Autodesk Inventor part; units mm, degrees
(part 2 of 3)
  measures "d1135" distance of L2.end L36.start
  measures "d1140" distance of L13.end A26.centre
  measures "d1141" distance from line of A2.centre L178
  measures "d1142" distance of L20.end L181.end
  measures "d1145" distance of A4.centre A28.centre
extrude "Extrusion27" add sketch "Sketch20" against normal blind 0.025 contours A0 L0 L8 A1 L7 L4 | A1 L32 L31 L30 | L41 A7 L40 L13 A6 | L9 A2 L10 A3 | A3 L177 L178 L179 | L45 L44 L43 A7 | L54 A9 L53 L13 A8 | L11 A38 A39 | A39 L402 L401 L400 | L58 L57 L56 A9 | L11 A36 L247 A37 L248 | A37 L253 L254 L255 | L67 A11 L66 L13 A10 | L71 L70 L69 A11 | L11 A41 L257 A40 L264 | A40 L257 L262 L266 | L80 A13 L79 L13 A12 | L84 L83 L82 A13 | L11 A43 L270 A42 L277 | A42 L270 L275 L279 | L93 A15 L92 L13 A14 | L97 L96 L95 A15 | L11 A45 L283 A44 L290 | A44 L283 L288 L292 | L106 A17 L105 L13 A16 | L110 L109 L108 A17 | L11 A47 L296 A46 L303 | A46 L296 L301 L305 | L119 A19 L118 L13 A18 | L123 L122 L121 A19 | L11 A49 L309 A48 L316 | A48 L309 L314 L318 | L132 A21 L131 L13 A20 | L136 L135 L134 A21 | L11 A51 L322 A50 L329 | A50 L322 L327 L331 | L145 A23 L144 L13 A22 | L149 L148 L147 A23 | L11 A53 L335 A52 L342 | A52 L335 L340 L344 | L158 A25 L157 L13 A24 | L162 L161 L160 A25 | L11 A55 L348 A54 L355 | A54 L348 L353 L357 | L171 A27 L170 L13 A26 | L175 L174 L173 A27 | L11 A57 L361 A56 L368 | A56 L361 L366 L370 | L22 A5 L28 L14 A4 | L182 L181 L180 A5 | L11 A59 L374 A58 L381 | A58 L374 L379 L383 | L186 A29 L192 L14 A28 | L196 L195 L194 A29 | L11 A61 L387 A60 L394 | A60 L387 L392 L396 | L200 A31 L206 L14 A30 | L210 L209 L208 A31 | L14 A34 L228 A35 L234 | A35 L238 L237 L236 | L214 A33 L220 L14 A32 | L224 L223 L222 A33
extrude "Extrusion28" add sketch "Sketch20" along normal blind 0.625 contours A0 L0 L8 A1 L7 L4 | L41 A7 L40 L13 A6 | L9 A2 L10 A3 | L54 A9 L53 L13 A8 | L11 A38 A39 | L11 A36 L247 A37 L248 | L67 A11 L66 L13 A10 | L11 A41 L257 A40 L264 | L80 A13 L79 L13 A12 | L11 A43 L270 A42 L277 | L93 A15 L92 L13 A14 | L11 A45 L283 A44 L290 | L106 A17 L105 L13 A16 | L11 A47 L296 A46 L303 | L119 A19 L118 L13 A18 | L11 A49 L309 A48 L316 | L132 A21 L131 L13 A20 | L11 A51 L322 A50 L329 | L145 A23 L144 L13 A22 | L11 A53 L335 A52 L342 | L158 A25 L157 L13 A24 | L11 A55 L348 A54 L355 | L171 A27 L170 L13 A26 | L11 A57 L361 A56 L368 | L22 A5 L28 L14 A4 | L11 A59 L374 A58 L381 | L186 A29 L192 L14 A28 | L11 A61 L387 A60 L394 | L200 A31 L206 L14 A30 | L14 A34 L228 A35 L234 | L214 A33 L220 L14 A32
sketch "Sketch15" plane through (0, 0, 0.6) normal (0, 0, 1) x (1, 0, 0)
  line L0 (-6.2, -4) -> (1.6, -4)
  line L1 (1.6, -4) -> (1.6, 4)
  line L2 (1.6, 4) -> (-6.2, 4)
  line L3 (-6.2, 4) -> (-6.2, -4)
  line L4 (-6.2, -4) -> (1.6, 4) construction
  line L5 (1.6, -4) -> (-6.2, 4) construction
  line L6 (-6.5, 4.3) -> (1.9, 4.3)
  line L7 (1.9, 4.3) -> (1.9, -4.3)
  line L8 (1.9, -4.3) -> (-6.5, -4.3)
  line L9 (-6.5, -4.3) -> (-6.5, 4.3)
  line L10 (-6.2, 4) -> (-6.5, 4)
  line L11 (-6.5, 4) -> (-6.5, 4.3)
  line L12 (-6.5, 4.3) -> (-6.2, 4.3)
  line L13 (-6.2, 4.3) -> (-6.2, 4)
  line L14 (1.6, 4) -> (1.9, 4)
  line L15 (1.9, 4) -> (1.9, 4.3)
  line L16 (1.9, 4.3) -> (1.6, 4.3)
  line L17 (1.6, 4.3) -> (1.6, 4)
  line L18 (1.6, -4) -> (1.9, -4)
  line L19 (1.9, -4) -> (1.9, -4.3)
  line L20 (1.9, -4.3) -> (1.6, -4.3)
  line L21 (1.6, -4.3) -> (1.6, -4)
  line L22 (-6.5, -4.3) -> (-6.2, -4.3)
  line L23 (-6.2, -4.3) -> (-6.2, -4)
  line L24 (-6.2, -4) -> (-6.5, -4)
  line L25 (-6.5, -4) -> (-6.5, -4.3)
  line L26 (-6.975, 4.775) -> (-6.975, 2.27) projected
  line L27 (-6.47, 4.775) -> (-6.975, 4.775) projected
  line L28 (-6.2975, -4.1) -> (1.6975, -4.1)
  line L29 (1.6975, -4.1) -> (1.6975, 4.1)
  line L30 (1.6975, 4.1) -> (-6.2975, 4.1)
  line L31 (-6.2975, 4.1) -> (-6.2975, -4.1)
  line L32 (-6.2975, -4.1) -> (1.6975, 4.1) construction
  line L33 (1.6975, -4.1) -> (-6.2975, 4.1) construction
  arc A0 (-6.975, -0.27) -> (-6.975, 0.27) centre (-6.975, 0) ccw projected
  point P0 (-2.3, 0)
  point P1 (-2.3, 0)
  point P2 (-6.705, 0)
  dimension "d952" = 7.8
  dimension "d953" = 8
  dimension "d954" = 0.3
  dimension "d961" = 0.475
  dimension "d962" = 0.475
  dimension "d966" = 0.1
  constraints: 64 end point, 14 parallel, 7 perpendicular, 6 horizontal, 5 midpoint, 1 horizontal alignment, 1 point on circle, 1 point on line, 3 other
  measures "d952" distance of L2.end L1.end
  measures "d953" distance of L1.end L0.end
  measures "d954" distance between parallel lines of L2 L6
  measures "d961" distance between parallel lines of L9 L26
  measures "d962" distance between parallel lines of L27 L6
  measures "d966" distance between parallel lines of L30 L2
extrude "Extrusion20" add sketch "Sketch15" along normal blind 1.55
fillet "Fillet4" radius 0.3 4 edges at (1.9, 0, 2.15) (-2.3, -4.3, 2.15) (-2.3, 4.3, 2.15) (-6.5, 0, 2.15)
extrude "Extrusion22" cut sketch "Sketch15" along normal through all contours L23 L28 L31 L24 | L18 L29 L28 L21 | L10 L31 L30 L13 | L23 L8 L9 L24 L31 L28 | L17 L30 L29 L14 | L18 L7 L8 L21 L28 L29 | L10 L9 L6 L13 L30 L31 | L29 L30 L17 L6 L7 L14
extrude "Extrusion23" cut sketch "Sketch15" along normal blind 1.4 contours L3 L2 L1 L0 | L24 L31 L10 L3 | L0 L21 L28 L23 | L23 L28 L31 L24 | L1 L14 L29 L18 | L18 L29 L28 L21 | L13 L30 L17 L2 | L10 L31 L30 L13 | L17 L30 L29 L14
fillet "Fillet5" radius 0.3 4 edges at (-2.3, -4.1, 2) (-6.2975, 0, 2) (-2.3, 4.1, 2) (1.6975, 0, 2)
extrude "Extrusion24" cut sketch "Sketch15" along normal blind 0.1 contours L3 L2 L1 L0 | L24 L31 L10 L3 | L0 L21 L28 L23 | L23 L28 L31 L24 | L1 L14 L29 L18 | L18 L29 L28 L21 | L13 L30 L17 L2 | L10 L31 L30 L13 | L28 L21 L8 L23 | L24 L9 L10 L31 | L17 L30 L29 L14 | L29 L14 L7 L18 | L13 L6 L17 L30
sketch "Sketch16" plane through (0, 0, 2.15) normal (0, 0, 1) x (1, 0, 0)
  line L0 (0.9007, -3.777) -> (-5.4993, -3.777)
  line L1 (-5.9993, -3.277) -> (-5.9993, 3.123)
  line L2 (-5.4993, 3.623) -> (0.9007, 3.623)
  line L3 (1.4007, 3.123) -> (1.4007, -3.277)
  line L4 (1.4007, -3.777) -> (-5.9993, 3.623) construction
  line L5 (-5.9993, -3.777) -> (1.4007, 3.623) construction
  arc A0 (-5.4993, 3.623) -> (-5.9993, 3.123) centre (-5.4993, 3.123) ccw
  arc A1 (1.4007, 3.123) -> (0.9007, 3.623) centre (0.9007, 3.123) ccw
  arc A2 (0.9007, -3.777) -> (1.4007, -3.277) centre (0.9007, -3.277) ccw
  arc A3 (-5.9993, -3.277) -> (-5.4993, -3.777) centre (-5.4993, -3.277) ccw
  point P0 (-2.2993, -0.077)
  point P1 (-2.2993, -0.077)
  dimension "d957" = 7.4
  dimension "d958" = 0.5
  constraints: 12 end point, 8 point on circle, 8 point on line, 8 tangent, 4 centre point, 3 equal radius, 2 parallel, 2 perpendicular, 1 coincident, 1 horizontal, 1 midpoint
  measures "d957" distance of L4.end L5.end
  measures "d958" radius of A0
extrude "Extrusion21" add sketch "Sketch16" along normal blind 0.1
sketch "Sketch18" plane through (0, 0, 2.25) normal (0, 0, 1) x (1, 0, 0)
  line L0 (0.9007, -3.777) -> (-5.4993, -3.777)
  line L1 (-5.9993, -3.277) -> (-5.9993, 3.123)
  line L2 (-5.4993, 3.623) -> (0.9007, 3.623)
  line L3 (1.4007, 3.123) -> (1.4007, -3.277)
  line L4 (1.4007, -3.777) -> (-5.9993, 3.623) construction
  line L5 (-5.9993, -3.777) -> (1.4007, 3.623) construction
  arc A0 (-5.4993, 3.623) -> (-5.9993, 3.123) centre (-5.4993, 3.123) ccw
  arc A1 (1.4007, 3.123) -> (0.9007, 3.623) centre (0.9007, 3.123) ccw
  arc A2 (0.9007, -3.777) -> (1.4007, -3.277) centre (0.9007, -3.277) ccw
  arc A3 (-5.9993, -3.277) -> (-5.4993, -3.777) centre (-5.4993, -3.277) ccw
  line L6 (-5.9993, -2.3578) -> (-4.5801, -3.777)
  line L7 (1.4007, -3.277) -> (1.4007, 3.123) projected
  line L8 (0.9007, 3.623) -> (-5.4993, 3.623) projected
  point P0 (-2.2993, -0.077)
  point P1 (-2.2993, -0.077)
  dimension "d972" = 7.4
  dimension "d973" = 0.5
  dimension "d976" = 45
  constraints: 14 end point, 10 point on line, 8 point on circle, 8 tangent, 4 centre point, 3 equal radius, 2 collinear, 2 parallel, 2 perpendicular, 1 coincident, 1 horizontal, 1 midpoint
  measures "d972" distance of L4.end L5.end
  measures "d973" radius of A0
  measures "d976" angle of L1 L6
extrude "Extrusion25" add sketch "Sketch18" along normal blind 0.001 contours L0 A3 L1 L6
sketch "Sketch17" plane through (0, 0, 2.25) normal (0, 0, 1) x (1, 0, 0)
  line L0 (-2.3072, -0.8881) -> (-2.4609, -0.8881)
  line L1 (-2.3072, -0.7289) -> (-2.3072, -0.8881)
  line L2 (-2.4609, -1.0504) -> (-2.1407, -1.0504)
  line L3 (-2.4668, -0.7289) -> (-2.3072, -0.7289)
  line L4 (-2.7903, -0.5636) -> (-2.7903, -0.7289)
  line L5 (-2.4668, -0.5636) -> (-2.4668, -0.7289)
  line L6 (-2.63, -0.5636) -> (-2.7903, -0.5636)
  line L7 (-2.63, -0.4013) -> (-2.7903, -0.4013)
  line L8 (-2.63, -0.4013) -> (-2.63, -0.5636)
  line L9 (-2.3072, -0.7289) -> (-2.3072, -0.5636)
  line L10 (-2.1407, -0.7289) -> (-2.3072, -0.7289)
  line L11 (-2.3072, -0.5636) -> (-2.1407, -0.5636)
  line L12 (-2.3072, -0.4013) -> (-2.4684, -0.4013)
  line L13 (-2.3072, -0.4013) -> (-2.3072, -0.5636)
  line L14 (-2.3072, -0.5636) -> (-2.4668, -0.5636)
  line L15 (-2.3037, -1.207) -> (-2.3037, -1.3643)
  line L16 (-4.4057, -1.2114) -> (-4.4057, -0.8881)
  line L17 (-4.0783, -1.2114) -> (-4.2447, -1.2114)
  line L18 (-4.5693, -1.2114) -> (-4.4057, -1.2114)
  line L19 (-4.2447, -1.2114) -> (-4.2447, -1.3643)
  line L20 (-4.2447, -1.3643) -> (-4.4057, -1.3643)
  line L21 (-4.0783, -1.3643) -> (-4.0783, -1.2114)
  line L22 (-3.9152, -1.3643) -> (-4.0783, -1.3643)
  line L23 (-4.2447, -1.5323) -> (-3.9212, -1.5323)
  line L24 (-3.9212, -1.5323) -> (-3.9212, -1.6965)
  line L25 (-4.2447, -1.6965) -> (-4.2447, -1.5323)
  line L26 (-4.5693, -1.6901) -> (-4.5693, -1.2114)
  line L27 (-4.4057, -1.3643) -> (-4.4057, -1.6901)
  line L28 (-4.4057, -1.6901) -> (-4.5693, -1.6901)
  line L29 (-3.2789, -0.8881) -> (-3.7606, -0.8881)
  line L30 (-3.6008, -1.0498) -> (-3.2789, -1.0498)
  line L31 (-3.6008, -1.2061) -> (-3.6008, -1.0498)
  line L32 (-3.2789, -1.2061) -> (-3.6008, -1.2061)
  line L33 (-3.7606, -1.2061) -> (-3.6008, -1.2061)
  line L34 (-3.7606, -0.8881) -> (-3.7606, -1.2061)
  line L35 (-3.2789, -1.3643) -> (-3.2789, -1.2061)
  line L36 (-3.6008, -1.3643) -> (-3.4396, -1.3643)
  line L37 (-3.6008, -1.2061) -> (-3.6008, -1.3643)
  line L38 (-3.9152, -0.8881) -> (-3.9152, -1.3643)
  line L39 (-3.4396, -1.3643) -> (-3.4396, -1.5272)
  line L40 (-3.439, -0.7259) -> (-3.6002, -0.7259)
  line L41 (-3.2789, -1.0498) -> (-3.2789, -0.8881)
  line L42 (-3.1151, -1.0498) -> (-3.2789, -1.0498)
  line L43 (-3.1151, -0.8881) -> (-3.1151, -1.0498)
  line L44 (-2.9507, -0.8881) -> (-3.1151, -0.8881)
  line L45 (-3.2789, -1.0498) -> (-3.2789, -1.2061)
  line L46 (-1.8231, -0.8881) -> (-1.6598, -0.8881)
  line L47 (-1.4972, -1.0504) -> (-1.8231, -1.0504)
  line L48 (-1.9819, -0.8881) -> (-2.1407, -0.8881)
  line L49 (-2.1407, -0.7289) -> (-2.1407, -0.8881)
  line L50 (-1.8231, -1.0504) -> (-1.8231, -0.8881)
  line L51 (-2.1407, -1.0504) -> (-2.1407, -1.207)
  line L52 (-1.9819, -1.207) -> (-1.9819, -0.8881)
  line L53 (-1.8231, -1.215) -> (-1.6598, -1.215)
  line L54 (-1.6598, -0.8881) -> (-1.6598, -0.7289)
  line L55 (-3.9212, -0.4013) -> (-3.9212, -0.5636)
  line L56 (-3.9212, -0.5636) -> (-4.0807, -0.5636)
  line L57 (-4.2425, -0.4013) -> (-3.9212, -0.4013)
  line L58 (-4.2447, -0.4013) -> (-4.4057, -0.4013)
  line L59 (-4.5665, -0.5636) -> (-4.2425, -0.5636)
  line L60 (-4.5665, -0.7259) -> (-4.5665, -0.5636)
  line L61 (-4.2395, -0.7259) -> (-4.5665, -0.7259)
  line L62 (-4.0807, -0.8881) -> (-3.9152, -0.8881)
  line L63 (-4.4057, -0.8881) -> (-4.2395, -0.8881)
  line L64 (-4.2395, -0.8881) -> (-4.2395, -0.7259)
  line L65 (-4.0807, -0.5636) -> (-4.0807, -0.8881)
  line L66 (-4.2425, -0.5636) -> (-4.2425, -0.4013)
  line L67 (-2.9501, -0.4013) -> (-2.9501, -0.7259)
  line L68 (-2.9501, -0.7259) -> (-3.1162, -0.7259)
  line L69 (-3.1162, -0.4013) -> (-2.9501, -0.4013)
  line L70 (-3.1162, -0.7259) -> (-3.1162, -0.5636)
  line L71 (-3.6002, -0.5628) -> (-3.439, -0.5628)
  line L72 (-3.6002, -0.7259) -> (-3.6002, -0.5628)
  line L73 (-3.439, -0.5628) -> (-3.439, -0.7259)
  line L74 (-3.1162, -0.5636) -> (-3.2789, -0.5636)
  line L75 (-3.2789, -0.5636) -> (-3.2789, -0.4013)
  line L76 (-3.9212, -1.6965) -> (-4.2447, -1.6965)
  line L77 (-4.2456, -2.1791) -> (-3.7554, -2.1791)
  line L78 (-4.4066, -2.0183) -> (-3.6011, -2.0183)
  line L79 (-4.2456, -2.6678) -> (-4.2456, -2.1791)
  line L80 (-4.5703, -1.8527) -> (-3.4399, -1.8527)
  line L81 (-4.4066, -2.8312) -> (-4.4066, -2.0183)
  line L82 (-3.7554, -2.1791) -> (-3.7554, -2.6678)
  line L83 (-3.7554, -2.6678) -> (-4.2456, -2.6678)
  line L84 (-4.5703, -2.982) -> (-4.5703, -1.8527)
  line L85 (-3.6011, -2.0183) -> (-3.6011, -2.8312)
  line L86 (-3.6011, -2.8312) -> (-4.4066, -2.8312)
  line L87 (-3.4399, -2.982) -> (-4.5703, -2.982)
  line L88 (-3.4399, -1.8527) -> (-3.4399, -2.982)
  line L89 (-2.7903, -0.7289) -> (-2.63, -0.7289)
  line L90 (-2.63, -0.7289) -> (-2.63, -1.207)
  line L91 (-2.9507, -1.2061) -> (-2.9507, -0.8881)
  line L92 (-2.4609, -0.8881) -> (-2.4609, -1.0504)
  line L93 (-2.9501, -1.8542) -> (-2.9501, -2.0183)
  line L94 (-2.9501, -2.1791) -> (-2.6293, -2.1791)
  line L95 (-2.7903, -1.8542) -> (-2.9501, -1.8542)
  line L96 (-2.9501, -2.0183) -> (-2.7903, -2.0183)
  line L97 (-2.7903, -2.0183) -> (-2.7903, -1.8542)
  line L98 (-2.63, -2.0183) -> (-2.63, -1.8542)
  line L99 (-2.7903, -1.6901) -> (-2.9507, -1.6901)
  line L100 (-2.7903, -1.6901) -> (-2.7903, -1.8542)
  line L101 (-2.9507, -1.5272) -> (-2.9507, -1.6901)
  line L102 (-2.7903, -1.8542) -> (-2.63, -1.8542)
  line L103 (-2.63, -1.5272) -> (-2.9507, -1.5272)
  line L104 (-2.9507, -1.8542) -> (-2.9507, -1.6901)
  line L105 (-3.2789, -1.2061) -> (-2.9507, -1.2061)
  line L106 (-3.2789, -1.3643) -> (-2.9507, -1.3643)
  line L107 (-3.7606, -1.5272) -> (-3.7606, -1.6901)
  line L108 (-3.4396, -1.5272) -> (-3.7606, -1.5272)
  line L109 (-3.7606, -1.6901) -> (-3.2789, -1.6901)
  line L110 (-3.2789, -1.5272) -> (-2.9507, -1.5272)
  line L111 (-3.2789, -1.5272) -> (-3.2789, -1.6901)
  line L112 (-3.1153, -2.0183) -> (-2.9501, -2.0183)
  line L113 (-3.1153, -1.8542) -> (-2.9507, -1.8542)
  line L114 (-2.9501, -2.0183) -> (-2.9501, -2.1791)
  line L115 (-2.9507, -1.6901) -> (-3.2789, -1.6901)
  line L116 (-3.2789, -1.6901) -> (-3.2789, -2.0183)
  line L117 (-3.1153, -2.1791) -> (-3.1153, -2.0183)
  line L118 (-3.2789, -2.0183) -> (-3.1153, -2.0183)
  line L119 (-3.1153, -2.0183) -> (-3.1153, -1.8542)
  line L120 (-1.1756, -0.4013) -> (-1.1756, -0.728)
  line L121 (-1.1766, -0.4013) -> (-1.3407, -0.4013)
  line L122 (-1.1741, -0.8881) -> (-0.5231, -0.8881)
  line L123 (-0.6864, -0.728) -> (-0.8486, -0.728)
  line L124 (-0.8486, -0.728) -> (-0.8486, -0.5636)
  line L125 (-0.8486, -0.5636) -> (-1.0117, -0.5636)
  line L126 (-0.8486, -0.5636) -> (-0.6864, -0.5636)
  line L127 (-0.6864, -0.5636) -> (-0.6864, -0.728)
  line L128 (-0.5231, -0.8881) -> (-0.5231, -0.4013)
  line L129 (-2.1407, -0.4013) -> (-2.1407, -0.5636)
  line L130 (-1.8231, -0.4013) -> (-2.1407, -0.4013)
  line L131 (-1.6598, -0.7289) -> (-1.3365, -0.7289)
  line L132 (-1.3365, -0.7289) -> (-1.3365, -0.5636)
  line L133 (-1.3365, -0.5636) -> (-1.8231, -0.5636)
  line L134 (-1.6598, -0.4013) -> (-1.8231, -0.4013)
  line L135 (-1.8231, -0.5636) -> (-1.8231, -0.4013)
  line L136 (-2.63, -1.2061) -> (-2.63, -1.3643)
  line L137 (-2.63, -1.3643) -> (-2.63, -1.5272)
  line L138 (-2.9507, -1.5272) -> (-2.9507, -1.3643)
  line L139 (-2.63, -1.3643) -> (-2.9507, -1.3643)
  line L140 (-2.9507, -1.2061) -> (-2.63, -1.2061)
  line L141 (-2.9507, -1.3643) -> (-2.9507, -1.2061)
  line L142 (-2.63, -1.207) -> (-2.3037, -1.207)
  line L143 (-2.4668, -1.3643) -> (-2.63, -1.3643)
  line L144 (-2.63, -1.8542) -> (-2.4668, -1.8542)
  line L145 (-2.4684, -1.6901) -> (-2.4684, -1.8542)
  line L146 (-2.63, -1.6901) -> (-2.4684, -1.6901)
  line L147 (-2.63, -1.8542) -> (-2.63, -1.6901)
  line L148 (-2.4684, -1.8542) -> (-2.3037, -1.8542)
  line L149 (-2.4668, -2.0183) -> (-2.63, -2.0183)
  line L150 (-2.4668, -1.8542) -> (-2.4668, -2.0183)
  line L151 (-2.6293, -2.338) -> (-2.4677, -2.338)
  line L152 (-2.6293, -2.1791) -> (-2.6293, -2.338)
  line L153 (-2.3037, -1.8542) -> (-2.3037, -2.1797)
  line L154 (-2.1407, -1.8542) -> (-1.9783, -1.8542)
  line L155 (-2.1407, -2.1797) -> (-2.1407, -1.8542)
  line L156 (-1.9783, -1.8542) -> (-1.9783, -2.1797)
  line L157 (-2.3008, -2.1797) -> (-2.4677, -2.1797)
  line L158 (-2.4677, -2.1797) -> (-2.4677, -2.338)
  line L159 (-2.3037, -2.1797) -> (-2.1407, -2.1797)
  line L160 (-2.3008, -2.338) -> (-2.3008, -2.1797)
  line L161 (-2.4677, -2.338) -> (-2.3008, -2.338)
  line L162 (-2.4677, -2.338) -> (-2.4677, -2.5032)
  line L163 (-2.4677, -2.5032) -> (-1.9776, -2.5032)
  line L164 (-1.4972, -1.6901) -> (-1.4972, -1.5272)
  line L165 (-1.4972, -1.5272) -> (-1.3365, -1.5272)
  line L166 (-1.3365, -1.5272) -> (-1.3365, -1.3643)
  line L167 (-1.3365, -1.3643) -> (-1.4972, -1.3643)
  line L168 (-1.4972, -1.3643) -> (-1.4972, -1.0504)
  line L169 (-0.3615, -0.5636) -> (-0.3615, -0.4013)
  line L170 (-0.0419, -0.5636) -> (0.1158, -0.5636)
  line L171 (-0.3615, -0.4013) -> (-0.0419, -0.4013)
  line L172 (-0.0419, -0.4013) -> (-0.0419, -0.5636)
  line L173 (-0.1998, -0.8881) -> (-0.1998, -1.0498)
  line L174 (-0.2017, -0.5636) -> (-0.3615, -0.5636)
  line L175 (-0.3615, -1.207) -> (-0.0419, -1.207)
  line L176 (-0.0419, -1.0498) -> (-0.0419, -1.207)
  line L177 (-0.2017, -0.728) -> (-0.2017, -0.5636)
  line L178 (-0.0419, -0.728) -> (-0.2017, -0.728)
  line L179 (-0.0419, -1.0498) -> (-0.1998, -1.0498)
  line L180 (-0.0419, -1.0507) -> (-0.0419, -0.728)
  line L181 (0.1158, -1.0507) -> (-0.0419, -1.0507)
  line L182 (0.1158, -0.5636) -> (0.1158, -1.0507)
  line L183 (-1.1741, -1.0498) -> (-1.1741, -0.8881)
  line L184 (-1.1756, -0.728) -> (-1.3361, -0.728)
  line L185 (-1.3361, -0.728) -> (-1.3361, -1.0498)
  line L186 (-1.0117, -1.0498) -> (-0.6878, -1.0498)
  line L187 (-1.0117, -1.207) -> (-1.0117, -1.0498)
  line L188 (-1.3361, -1.0498) -> (-1.1741, -1.0498)
  line L189 (-1.3365, -1.3643) -> (-0.3615, -1.3643)
  line L190 (-1.3365, -1.3643) -> (-1.3365, -1.207)
  line L191 (-1.3365, -1.207) -> (-1.0117, -1.207)
  line L192 (-0.6878, -1.0498) -> (-0.6878, -1.207)
  line L193 (-0.6878, -1.207) -> (-0.5231, -1.207)
  line L194 (-0.5231, -1.207) -> (-0.5231, -0.8881)
  line L195 (-0.5231, -0.8881) -> (-0.1998, -0.8881)
  line L196 (-0.3615, -1.207) -> (-0.3615, -1.3643)
  line L197 (-0.1997, -1.3643) -> (-0.3615, -1.3643)
  line L198 (0.1158, -1.3707) -> (-0.0419, -1.3707)
  line L199 (-0.0419, -1.3707) -> (-0.0419, -1.5323)
  line L200 (-0.1997, -1.5323) -> (-0.1997, -1.3643)
  line L201 (-0.0419, -1.5323) -> (-0.1997, -1.5323)
  line L202 (-0.3615, -1.3643) -> (-0.3615, -1.5323)
  line L203 (-0.3615, -1.5323) -> (-0.1997, -1.5323)
  line L204 (0.1158, -1.6965) -> (0.1158, -1.3707)
  line L205 (-0.1997, -1.6965) -> (0.1158, -1.6965)
  line L206 (-0.1997, -1.5323) -> (-0.1997, -1.6965)
  line L207 (-2.1407, -1.5322) -> (-2.4668, -1.5322)
  line L208 (-2.4668, -1.5322) -> (-2.4668, -1.3643)
  line L209 (-2.1407, -1.207) -> (-1.9819, -1.207)
  line L210 (-2.1407, -1.3643) -> (-2.1407, -1.5322)
  line L211 (-2.1407, -1.5323) -> (-1.9792, -1.5323)
  line L212 (-2.1407, -1.6965) -> (-2.1407, -1.5323)
  line L213 (-1.8231, -1.5323) -> (-1.8231, -1.215)
  line L214 (-1.9792, -1.5323) -> (-1.9792, -1.6965)
  line L215 (-1.9792, -1.6965) -> (-2.1407, -1.6965)
  line L216 (-1.6598, -1.215) -> (-1.6598, -1.5323)
  line L217 (-1.6598, -1.5323) -> (-1.8231, -1.5323)
  line L218 (-2.3037, -1.3643) -> (-2.1407, -1.3643)
  line L219 (-1.0145, -1.5323) -> (-0.8508, -1.5323)
  line L220 (-1.0145, -1.6965) -> (-1.0145, -1.5323)
  line L221 (-0.8508, -1.6965) -> (-1.0145, -1.6965)
  line L222 (-0.8508, -1.5323) -> (-0.8508, -1.6965)
  line L223 (-0.3615, -1.5323) -> (-0.5251, -1.5323)
  line L224 (-0.3615, -1.6965) -> (-0.3615, -1.5323)
  line L225 (-0.5251, -1.5323) -> (-0.5251, -1.6965)
  line L226 (-0.5251, -1.6965) -> (-0.3615, -1.6965)
  line L227 (-1.6598, -1.8542) -> (-1.6598, -1.6901)
  line L228 (-1.8231, -1.8542) -> (-1.6598, -1.8542)
  line L229 (-1.6598, -1.6901) -> (-1.4972, -1.6901)
  line L230 (-1.8231, -2.1797) -> (-1.8231, -1.8542)
  line L231 (-1.6598, -2.0197) -> (-1.6598, -1.8542)
  line L232 (-1.6598, -1.8542) -> (-1.4982, -1.8542)
  line L233 (-1.4982, -2.0197) -> (-1.6598, -2.0197)
  line L234 (-1.4982, -1.8542) -> (-1.4982, -2.0197)
  line L235 (-1.3407, -2.1791) -> (-1.3407, -1.6965)
  line L236 (-1.1766, -2.1791) -> (-1.3407, -2.1791)
  line L237 (-1.1766, -1.6965) -> (-1.1766, -2.1791)
  line L238 (-1.3407, -1.6965) -> (-1.1766, -1.6965)
  line L239 (-0.6878, -2.6678) -> (-0.6878, -2.1791)
  line L240 (-0.8488, -2.8312) -> (-0.8488, -2.0183)
  line L241 (-0.6878, -2.1791) -> (-0.1976, -2.1791)
  line L242 (-1.0124, -2.982) -> (-1.0124, -1.8527)
  line L243 (-0.8488, -2.0183) -> (-0.0433, -2.0183)
  line L244 (-1.0124, -1.8527) -> (0.1179, -1.8527)
  line L245 (-0.1976, -2.6678) -> (-0.6878, -2.6678)
  line L246 (-0.0433, -2.8312) -> (-0.8488, -2.8312)
  line L247 (0.1179, -2.982) -> (-1.0124, -2.982)
  line L248 (-0.0433, -2.0183) -> (-0.0433, -2.8312)
  line L249 (0.1179, -1.8527) -> (0.1179, -2.982)
  line L250 (-0.1976, -2.1791) -> (-0.1976, -2.6678)
  line L251 (-1.8224, -2.5032) -> (-1.8224, -2.3411)
  line L252 (-1.9783, -2.1797) -> (-1.8231, -2.1797)
  line L253 (-1.3358, -2.6655) -> (-1.4972, -2.6655)
  line L254 (-1.4972, -2.6655) -> (-1.4972, -2.3392)
  line L255 (-1.3358, -2.4956) -> (-1.3358, -2.6655)
  line L256 (-1.1745, -2.4956) -> (-1.3358, -2.4956)
  line L257 (-1.1745, -2.3392) -> (-1.1745, -2.4956)
  line L258 (-1.4972, -2.3392) -> (-1.1745, -2.3392)
  line L259 (-2.1401, -2.988) -> (-2.1401, -2.8267)
  line L260 (-1.6547, -2.3411) -> (-1.6547, -2.5032)
  line L261 (-1.8224, -2.3411) -> (-1.6547, -2.3411)
  line L262 (-1.6547, -2.5032) -> (-1.8224, -2.5032)
  line L263 (-1.9776, -2.8267) -> (-1.9776, -2.5032)
  line L264 (-1.8225, -2.8267) -> (-1.8225, -2.6655)
  line L265 (-1.8225, -2.8267) -> (-1.8225, -2.988)
  line L266 (-1.6598, -2.8267) -> (-1.8225, -2.8267)
  line L267 (-1.8225, -2.6655) -> (-1.4972, -2.6655)
  line L268 (-1.6598, -2.9879) -> (-1.6598, -2.8267)
  line L269 (-1.4972, -2.9879) -> (-1.4972, -2.6655)
  line L270 (-1.4972, -2.9879) -> (-1.6598, -2.9879)
  line L271 (-1.8225, -2.988) -> (-2.1401, -2.988)
  line L272 (-1.8225, -2.8267) -> (-1.9776, -2.8267)
  line L273 (-2.4677, -2.6678) -> (-2.4677, -2.8267)
  line L274 (-2.4677, -2.8267) -> (-2.6293, -2.8267)
  line L275 (-2.3031, -2.6678) -> (-2.4677, -2.6678)
  line L276 (-2.3031, -2.8267) -> (-2.3031, -2.6678)
  line L277 (-2.1401, -2.8267) -> (-2.3031, -2.8267)
  line L278 (-2.6293, -2.8267) -> (-2.6293, -2.9902)
  line L279 (-3.2789, -2.5032) -> (-3.2789, -2.3411)
  line L280 (-3.2789, -2.3411) -> (-3.1153, -2.3411)
  line L281 (-3.1153, -2.5032) -> (-3.2789, -2.5032)
  line L282 (-3.1153, -2.3411) -> (-3.1153, -2.5032)
  line L283 (-2.9501, -2.1791) -> (-3.1153, -2.1791)
  line L284 (-2.9501, -2.1791) -> (-2.9501, -2.5032)
  line L285 (-2.9501, -2.5032) -> (-3.1153, -2.5032)
  line L286 (-3.1153, -2.5032) -> (-3.1153, -2.6678)
  line L287 (-3.1153, -2.6678) -> (-2.9501, -2.6678)
  line L288 (-3.2789, -2.6678) -> (-3.1153, -2.6678)
  line L289 (-2.9501, -2.6678) -> (-2.9501, -2.8267)
  line L290 (-2.9501, -2.8267) -> (-3.1153, -2.8267)
  line L291 (-3.1153, -2.8267) -> (-3.1153, -2.6678)
  line L292 (-2.7897, -2.8267) -> (-2.7897, -2.6678)
  line L293 (-3.2789, -2.9902) -> (-3.2789, -2.6678)
  line L294 (-2.6293, -2.9902) -> (-3.2789, -2.9902)
  line L295 (-2.7897, -2.6678) -> (-2.6293, -2.6678)
  line L296 (-2.6293, -2.6678) -> (-2.6293, -2.8267)
  line L297 (-2.6293, -2.8267) -> (-2.7897, -2.8267)
  line L298 (-2.7892, -0.0749) -> (-3.2789, -0.0749)
  line L299 (-3.2789, -0.2382) -> (-3.1162, -0.2382)
  line L300 (-3.2789, 0.0851) -> (-3.1162, 0.0851)
  line L301 (-3.4396, 0.2469) -> (-3.2789, 0.2469)
  line L302 (-3.2789, 0.2469) -> (-3.2789, 0.0851)
  line L303 (-2.7892, 0.0851) -> (-2.7892, -0.0749)
  line L304 (-2.7892, 0.0851) -> (-2.9501, 0.0851)
  line L305 (-2.7892, 0.2469) -> (-2.7892, 0.0851)
  line L306 (-2.9501, 0.2469) -> (-2.7892, 0.2469)
  line L307 (-3.4396, 0.0858) -> (-3.4396, 0.2469)
  line L308 (-2.6272, 0.8883) -> (-2.6272, 0.5766)
  line L309 (-2.787, 0.8883) -> (-2.6272, 0.8883)
  line L310 (-2.787, 0.7257) -> (-2.9501, 0.7257)
  line L311 (-2.9501, 0.5766) -> (-2.9501, 0.7257)
  line L312 (-3.1153, 0.5766) -> (-2.9501, 0.5766)
  line L313 (-2.9501, 0.7257) -> (-3.1153, 0.7257)
  line L314 (-3.1153, 0.7257) -> (-3.1153, 0.5766)
  line L315 (-3.1162, 0.4087) -> (-3.2789, 0.4087)
  line L316 (-3.2789, 0.4087) -> (-3.2789, 0.8883)
  line L317 (-2.9501, 1.051) -> (-2.7892, 1.051)
  line L318 (-2.9501, 0.7257) -> (-2.9501, 1.051)
  line L319 (-3.2789, 0.8883) -> (-3.1162, 0.8883)
  line L320 (-3.1162, 0.8883) -> (-3.1162, 1.051)
  line L321 (-2.787, 0.7257) -> (-2.787, 0.8883)
  line L322 (-2.5758, 2.4776) -> (-2.7083, 2.4776)
  line L323 (-2.5758, 2.4776) -> (-2.4465, 2.4776)
  line L324 (-2.5758, 2.6104) -> (-2.5758, 2.4776)
  line L325 (-2.7083, 2.6104) -> (-2.7083, 2.4776)
  line L326 (-2.9851, 2.8765) -> (-3.119, 2.8765)
  line L327 (-3.119, 2.8765) -> (-3.119, 2.7372)
  line L328 (-2.9851, 2.7372) -> (-2.9851, 2.8765)
  line L329 (-2.7083, 2.6104) -> (-2.5758, 2.6104)
  line L330 (-2.9851, 3.0109) -> (-2.9851, 2.8765)
  line L331 (-2.4465, 2.6098) -> (-2.5758, 2.6098)
  line L332 (-2.9851, 2.8765) -> (-2.5758, 2.8765)
  line L333 (-2.5758, 2.6098) -> (-2.5758, 2.8765)
  line L334 (-2.4465, 2.8765) -> (-2.4465, 2.6098)
  line L335 (-2.5758, 2.8765) -> (-2.4465, 2.8765)
  line L336 (-2.5758, 2.8765) -> (-2.5758, 3.0109)
  line L337 (-2.5758, 3.0109) -> (-2.9851, 3.0109)
  line L338 (-3.119, 2.7372) -> (-2.9851, 2.7372)
  line L339 (-3.119, 2.3469) -> (-3.119, 2.2076)
  line L340 (-2.9851, 2.3469) -> (-3.119, 2.3469)
  line L341 (-3.119, 2.2076) -> (-2.9851, 2.2076)
  line L342 (-2.9851, 2.2076) -> (-2.9851, 2.3469)
  line L343 (-2.9851, 2.2076) -> (-2.9851, 2.0832)
  line L344 (-2.9851, 2.0832) -> (-2.5758, 2.0832)
  line L345 (-2.5758, 2.0832) -> (-2.5758, 2.2076)
  line L346 (-2.5758, 2.2076) -> (-2.9851, 2.2076)
  line L347 (-2.4684, -0.2382) -> (-2.7903, -0.2382)
  line L348 (-2.7903, -0.2382) -> (-2.7903, -0.4013)
  line L349 (-3.1162, -0.2382) -> (-3.1162, -0.4013)
  line L350 (-2.4684, -0.4013) -> (-2.4684, -0.2382)
  line L351 (-2.4665, -0.0749) -> (-2.6293, -0.0749)
  line L352 (-2.3072, -0.2382) -> (-2.4665, -0.2382)
  line L353 (-2.4665, -0.2382) -> (-2.4665, -0.0749)
  line L354 (-2.3072, -0.0749) -> (-2.3072, -0.2382)
  line L355 (-2.4677, 0.5766) -> (-2.4677, 0.7277)
  line L356 (-3.1162, 0.0851) -> (-3.1162, 0.4087)
  line L357 (-2.9501, 0.0851) -> (-2.9501, 0.2469)
  line L358 (-2.7892, 0.0851) -> (-2.6293, 0.0851)
  line L359 (-2.6293, -0.0749) -> (-2.6293, 0.0851)
  line L360 (-2.4665, 0.2487) -> (-2.4665, -0.0749)
  line L361 (-2.4665, -0.0749) -> (-2.3072, -0.0749)
  line L362 (-2.6272, 0.5766) -> (-2.4677, 0.5766)
  line L363 (-3.1153, 1.5386) -> (-2.7892, 1.5386)
  line L364 (-3.1162, 1.5386) -> (-3.2789, 1.5386)
  line L365 (-3.2789, 1.5386) -> (-3.2789, 1.7042)
  line L366 (-3.2789, 1.7042) -> (-3.1162, 1.7042)
  line L367 (-3.1162, 1.7042) -> (-3.1162, 1.5386)
  line L368 (-2.63, 1.7042) -> (-2.63, 1.051)
  line L369 (-2.4679, 1.2133) -> (-2.4679, 1.5386)
  line L370 (-2.7892, 1.3778) -> (-2.7892, 1.5386)
  line L371 (-3.1153, 1.3778) -> (-3.1153, 1.5386)
  line L372 (-3.1153, 1.3778) -> (-2.9501, 1.3778)
  line L373 (-3.2789, 1.3778) -> (-3.1153, 1.3778)
  line L374 (-2.9501, 1.2144) -> (-3.1153, 1.2144)
  line L375 (-2.9501, 1.3778) -> (-2.9501, 1.2144)
  line L376 (-3.2789, 1.3778) -> (-3.2789, 1.2144)
  line L377 (-3.1153, 1.2144) -> (-3.1153, 1.3778)
  line L378 (-2.7892, 1.051) -> (-2.7892, 1.3778)
  line L379 (-3.2789, 1.051) -> (-3.2789, 1.2144)
  line L380 (-3.1162, 1.051) -> (-3.2789, 1.051)
  line L381 (-4.2447, -0.2382) -> (-4.2447, -0.4013)
  line L382 (-4.0817, -0.0749) -> (-4.0817, -0.2382)
  line L383 (-4.0817, -0.2382) -> (-3.7606, -0.2382)
  line L384 (-3.7606, -0.0749) -> (-3.9212, -0.0749)
  line L385 (-3.6002, 0.0858) -> (-3.4396, 0.0858)
  line L386 (-3.6002, -0.0749) -> (-3.6002, 0.0858)
  line L387 (-3.2789, -0.0749) -> (-3.2789, -0.2382)
  line L388 (-3.4396, -0.2382) -> (-3.4396, -0.0749)
  line L389 (-3.4396, -0.0749) -> (-3.6002, -0.0749)
  line L390 (-3.6002, -0.2382) -> (-3.4396, -0.2382)
  line L391 (-3.6002, -0.4013) -> (-3.2789, -0.4013)
  line L392 (-3.7606, -0.2382) -> (-3.7606, -0.0749)
  line L393 (-3.6002, -0.4013) -> (-3.6002, -0.2382)
  line L394 (-3.3988, 3.0109) -> (-3.2614, 3.0109)
  line L395 (-3.3988, 2.8765) -> (-3.531, 2.8765)
  line L396 (-3.531, 2.7431) -> (-3.531, 2.4776)
  line L397 (-3.6659, 2.4776) -> (-3.6659, 2.7431)
  line L398 (-3.531, 2.4776) -> (-3.6659, 2.4776)
  line L399 (-3.9386, 2.0832) -> (-3.9386, 3.0109)
  line L400 (-3.2614, 3.0109) -> (-3.2614, 2.0832)
  line L401 (-3.7988, 2.7431) -> (-3.7988, 2.0832)
  line L402 (-3.3988, 2.0832) -> (-3.3988, 2.7431)
  line L403 (-3.7988, 2.0832) -> (-3.9386, 2.0832)
  line L404 (-3.2614, 2.0832) -> (-3.3988, 2.0832)
  line L405 (-3.531, 2.7431) -> (-3.3988, 2.7431)
  line L406 (-3.6659, 2.7431) -> (-3.531, 2.7431)
  line L407 (-3.531, 2.8765) -> (-3.531, 2.7431)
  line L408 (-3.3988, 2.8765) -> (-3.3988, 3.0109)
  line L409 (-3.6659, 2.7431) -> (-3.7988, 2.7431)
  line L410 (-3.7988, 2.8765) -> (-3.6659, 2.8765)
  line L411 (-3.7988, 3.0109) -> (-3.7988, 2.8765)
  line L412 (-3.9386, 3.0109) -> (-3.7988, 3.0109)
  line L413 (-3.6659, 2.8765) -> (-3.6659, 2.7431)
  line L414 (-3.4406, 0.4126) -> (-3.4406, 0.2469)
  line L415 (-3.4406, 0.2469) -> (-3.9212, 0.2469)
  line L416 (-3.4406, 0.4126) -> (-4.0817, 0.4126)
  line L417 (-4.4057, -0.4013) -> (-4.4057, -0.2382)
  line L418 (-4.4057, -0.2382) -> (-4.2447, -0.2382)
  line L419 (-4.2447, -0.0749) -> (-4.0817, -0.0749)
  line L420 (-4.4066, 0.4087) -> (-4.2447, 0.4087)
  line L421 (-4.2447, 0.4087) -> (-4.2447, 0.2487)
  line L422 (-4.2447, 0.2487) -> (-4.4066, 0.2487)
  line L423 (-4.4066, 0.2487) -> (-4.4066, 0.4087)
  line L424 (-4.0817, 0.4126) -> (-4.0817, 0.0851)
  line L425 (-4.5693, 0.0847) -> (-4.4057, 0.0847)
  line L426 (-3.9212, -0.0749) -> (-3.9212, 0.2469)
  line L427 (-4.5693, -0.0772) -> (-4.5693, 0.0847)
  line L428 (-4.4057, -0.0772) -> (-4.5693, -0.0772)
  line L429 (-4.4057, 0.0847) -> (-4.4057, -0.0772)
  line L430 (-4.2447, 0.0851) -> (-4.2447, -0.0749)
  line L431 (-4.0817, 0.0851) -> (-4.2447, 0.0851)
  line L432 (-3.7545, 0.8891) -> (-4.2447, 0.8891)
  line L433 (-3.6002, 0.7257) -> (-4.4057, 0.7257)
  line L434 (-4.5693, 0.5749) -> (-4.4057, 0.5749)
  line L435 (-3.439, 0.5749) -> (-4.5693, 0.5749)
  line L436 (-3.7545, 1.3778) -> (-3.7545, 0.8891)
  line L437 (-4.2447, 0.8891) -> (-4.2447, 1.3778)
  line L438 (-4.2447, 1.3778) -> (-3.7545, 1.3778)
  line L439 (-4.4057, 0.7257) -> (-4.4057, 1.5386)
  line L440 (-4.4057, 1.5386) -> (-3.6002, 1.5386)
  line L441 (-4.5693, 0.5749) -> (-4.5693, 1.7042)
  line L442 (-4.5693, 1.7042) -> (-3.439, 1.7042)
  line L443 (-3.439, 1.7042) -> (-3.439, 0.5749)
  line L444 (-3.6002, 1.5386) -> (-3.6002, 0.7257)
  line L445 (-4.4865, 2.2076) -> (-4.4865, 2.0832)
  line L446 (-4.3527, 2.2076) -> (-4.4865, 2.2076)
  line L447 (-4.3527, 2.2076) -> (-4.3527, 2.8765)
  line L448 (-4.4865, 2.0832) -> (-4.085, 2.0832)
  line L449 (-4.085, 2.0832) -> (-4.085, 2.2076)
  line L450 (-4.085, 2.2076) -> (-4.2124, 2.2076)
  line L451 (-4.2124, 2.8765) -> (-4.2124, 2.2076)
  line L452 (-4.4865, 2.8765) -> (-4.4865, 3.0109)
  line L453 (-4.3527, 2.8765) -> (-4.4865, 2.8765)
  line L454 (-4.085, 2.8765) -> (-4.2124, 2.8765)
  line L455 (-4.085, 3.0109) -> (-4.085, 2.8765)
  line L456 (-4.4865, 3.0109) -> (-4.085, 3.0109)
  line L457 (-4.6489, 2.4776) -> (-4.6489, 2.2076)
  line L458 (-4.7833, 2.6098) -> (-4.7833, 2.4776)
  line L459 (-4.7833, 2.2076) -> (-4.7833, 2.4776)
  line L460 (-4.7833, 2.0832) -> (-4.7833, 2.2076)
  line L461 (-4.6489, 2.2076) -> (-4.7833, 2.2076)
  line L462 (-5.1778, 2.4776) -> (-5.1778, 2.6098)
  line L463 (-4.7833, 2.4776) -> (-5.1778, 2.4776)
  line L464 (-4.7833, 2.2076) -> (-5.31, 2.2076)
  line L465 (-5.31, 2.0832) -> (-4.7833, 2.0832)
  line L466 (-5.31, 2.2076) -> (-5.31, 2.0832)
  line L467 (-4.7833, 2.4776) -> (-4.6489, 2.4776)
  line L468 (-5.1778, 2.6098) -> (-4.7833, 2.6098)
  line L469 (-5.31, 2.6098) -> (-5.1778, 2.6098)
  line L470 (-4.6489, 3.0109) -> (-4.6489, 2.8765)
  line L471 (-4.6489, 2.8765) -> (-5.1778, 2.8765)
  line L472 (-5.1778, 3.0109) -> (-4.6489, 3.0109)
  line L473 (-5.1778, 2.6098) -> (-5.1778, 2.8765)
  line L474 (-5.31, 2.8765) -> (-5.31, 2.6098)
  line L475 (-5.1778, 2.8765) -> (-5.31, 2.8765)
  line L476 (-5.1778, 2.8765) -> (-5.1778, 3.0109)
  line L477 (-1.8231, 0.4087) -> (-1.8231, 0.2487)
  line L478 (-1.8231, 0.2487) -> (-1.6598, 0.2487)
  line L479 (-1.4976, 0.5749) -> (-1.8224, 0.5749)
  line L480 (-1.8231, 0.2487) -> (-1.9771, 0.2487)
  line L481 (-1.9771, 0.2487) -> (-1.9771, 0.4087)
  line L482 (-1.9771, 0.4087) -> (-1.8231, 0.4087)
  line L483 (-1.9771, 0.4087) -> (-1.9771, 0.5766)
  line L484 (-1.1766, -0.2382) -> (-1.1766, -0.4013)
  line L485 (-1.3407, -0.2382) -> (-1.1766, -0.2382)
  line L486 (-1.3407, -0.4013) -> (-1.3407, -0.2382)
  line L487 (-1.0117, -0.4013) -> (-1.1756, -0.4013)
  line L488 (-0.6859, -0.2382) -> (-0.8488, -0.2382)
  line L489 (-0.6864, -0.2377) -> (-0.6864, -0.4013)
  line L490 (-0.6864, -0.4013) -> (-0.8486, -0.4013)
  line L491 (-0.8486, -0.4013) -> (-0.8486, -0.5636)
  line L492 (-1.0117, -0.5636) -> (-1.0117, -0.4013)
  line L493 (-0.6859, -0.0772) -> (-0.6859, -0.2382)
  line L494 (-0.8488, -0.2382) -> (-0.8488, -0.0772)
  line L495 (-0.8488, -0.0772) -> (-0.6859, -0.0772)
  line L496 (-0.6878, 0.0858) -> (-0.6878, -0.0785)
  line L497 (-0.8488, 0.0858) -> (-0.6878, 0.0858)
  line L498 (-1.0116, -0.0785) -> (-1.1745, -0.0785)
  line L499 (-1.0116, 0.0858) -> (-1.0116, -0.0785)
  line L500 (-1.1745, -0.0785) -> (-1.1745, 0.0858)
  line L501 (-1.1745, 0.0858) -> (-1.0116, 0.0858)
  line L502 (-1.1745, 0.0858) -> (-1.1745, 0.2487)
  line L503 (-0.8488, 0.2487) -> (-0.8488, 0.0858)
  line L504 (-0.6878, -0.0785) -> (-0.5231, -0.0785)
  line L505 (-0.5216, -0.0774) -> (-0.5216, -0.2377)
  line L506 (-0.5216, -0.2377) -> (-0.6864, -0.2377)
  line L507 (-0.5231, -0.4013) -> (-0.3615, -0.4013)
  line L508 (-0.3615, -0.4013) -> (-0.3615, -0.0774)
  line L509 (0.1158, -0.4013) -> (-0.0419, -0.4013)
  line L510 (-0.0419, -0.4013) -> (-0.0419, -0.0749)
  line L511 (0.1158, -0.0749) -> (0.1158, -0.4013)
  line L512 (-0.0419, -0.0749) -> (0.1158, -0.0749)
  line L513 (-0.3615, -0.0774) -> (-0.5216, -0.0774)
  line L514 (-0.1998, -0.0749) -> (-0.0419, -0.0749)
  line L515 (-0.1998, 0.0859) -> (-0.1998, -0.0749)
  line L516 (-0.3615, 0.0859) -> (-0.1998, 0.0859)
  line L517 (-0.5231, 0.2487) -> (-0.5231, -0.0785)
  line L518 (-0.3615, 0.2487) -> (-0.5231, 0.2487)
  line L519 (-0.3615, 0.2487) -> (-0.3615, 0.0859)
  line L520 (-0.0419, -0.0749) -> (-0.0419, 0.2487)
  line L521 (-0.0419, 0.2487) -> (-0.3615, 0.2487)
  line L522 (-1.6598, -0.2382) -> (-1.6598, -0.4013)
  line L523 (-1.6598, -0.0772) -> (-1.4982, -0.0772)
  line L524 (-1.8231, -0.2382) -> (-1.6598, -0.2382)
  line L525 (-1.6547, 0.4087) -> (-1.6547, 0.2487)
  line L526 (-1.6598, 0.2487) -> (-1.6598, 0.0847)
  line L527 (-1.8231, 0.0847) -> (-1.8231, 0.2487)
  line L528 (-1.6598, 0.0847) -> (-1.8231, 0.0847)
  line L529 (-1.8231, -0.4013) -> (-1.8231, -0.2382)
  line L530 (-1.4982, 0.0847) -> (-1.6598, 0.0847)
  line L531 (-1.3387, 0.4087) -> (-1.6547, 0.4087)
  line L532 (-1.6598, 0.0847) -> (-1.6598, -0.0772)
  line L533 (-1.4982, -0.0772) -> (-1.4982, 0.0847)
  line L534 (-1.3387, 0.2487) -> (-1.3387, 0.0858)
  line L535 (-1.3387, 0.0858) -> (-1.1745, 0.0858)
  line L536 (-1.6547, 0.2487) -> (-1.3387, 0.2487)
  line L537 (-0.3615, 0.5757) -> (-0.3615, 0.2487)
  line L538 (-0.5231, 0.7257) -> (-0.3615, 0.7257)
  line L539 (-0.3615, 0.7257) -> (-0.3615, 0.8883)
  line L540 (-0.2024, 0.8883) -> (-0.2024, 0.7288)
  line L541 (-0.2024, 0.5757) -> (-0.3615, 0.5757)
  line L542 (-0.2024, 0.5757) -> (-0.2024, 0.4086)
  line L543 (-0.2024, 0.7288) -> (-0.0488, 0.7288)
  line L544 (-0.0488, 0.7288) -> (-0.0488, 0.5671)
  line L545 (-0.0488, 0.4086) -> (-0.0488, 0.5671)
  line L546 (-0.2024, 0.4086) -> (-0.0488, 0.4086)
  line L547 (-1.3387, 1.051) -> (-0.8488, 1.051)
  line L548 (-1.4976, 0.7257) -> (-1.3387, 0.7257)
  line L549 (-1.4976, 0.5749) -> (-1.4976, 0.7257)
  line L550 (-1.0124, 0.5749) -> (-1.0124, 0.7257)
  line L551 (-1.0124, 0.7257) -> (-0.8508, 0.7257)
  line L552 (-1.1745, 0.4087) -> (-1.1745, 0.8883)
  line L553 (-0.6878, 0.8883) -> (-1.1745, 0.8883)
  line L554 (-0.8508, 0.5749) -> (-1.0124, 0.5749)
  line L555 (-0.8508, 0.7257) -> (-0.8508, 0.5749)
  line L556 (-0.5231, 0.7257) -> (-0.5231, 0.8883)
  line L557 (-0.6878, 0.8883) -> (-0.6878, 0.4087)
  line L558 (-1.1745, 0.4087) -> (-0.6878, 0.4087)
  line L559 (-1.1745, 0.2487) -> (-0.8488, 0.2487)
  line L560 (-1.3387, 0.7257) -> (-1.3387, 0.4087)
  line L561 (-1.9819, 1.051) -> (-1.9819, 1.2133)
  line L562 (-1.9819, 1.2133) -> (-2.4679, 1.2133)
  line L563 (-1.8224, 1.051) -> (-1.9819, 1.051)
  line L564 (-1.8224, 0.8883) -> (-1.8224, 1.051)
  line L565 (-2.3031, 0.2487) -> (-2.4665, 0.2487)
  line L566 (-2.3059, 1.051) -> (-2.3059, 0.8883)
  line L567 (-2.3059, 0.8883) -> (-1.8224, 0.8883)
  line L568 (-1.8224, 0.5749) -> (-1.8224, 0.8888)
  line L569 (-2.63, 1.051) -> (-2.3059, 1.051)
  line L570 (-2.3028, 0.7277) -> (-2.3028, 0.5766)
  line L571 (-2.4677, 0.7277) -> (-2.3028, 0.7277)
  line L572 (-2.3028, 0.5766) -> (-1.9771, 0.5766)
  line L573 (-2.3031, 0.4087) -> (-2.3031, 0.2487)
  line L574 (-2.3031, 0.4087) -> (-1.9771, 0.4087)
  line L575 (-1.0117, 1.2133) -> (-1.0117, 1.5386)
  line L576 (-0.8488, 1.051) -> (-0.8488, 1.2144)
  line L577 (-0.8488, 1.2144) -> (-0.6859, 1.2144)
  line L578 (-0.3615, 0.8883) -> (-0.2024, 0.8883)
  line L579 (-0.5231, 1.051) -> (-0.5231, 0.8883)
  line L580 (-0.6859, 1.051) -> (-0.5231, 1.051)
  line L581 (-0.6859, 1.2144) -> (-0.6859, 1.051)
  line L582 (-1.8224, 1.2133) -> (-1.9819, 1.2133)
  line L583 (-1.9819, 1.2133) -> (-1.9819, 1.5386)
  line L584 (-1.6598, 1.2133) -> (-1.6598, 1.051)
  line L585 (-1.6598, 1.051) -> (-1.4982, 1.051)
  line L586 (-1.8224, 0.8888) -> (-1.3387, 0.8888)
  line L587 (-1.8224, 1.5386) -> (-1.8224, 1.2133)
  line L588 (-1.3387, 0.8888) -> (-1.3387, 1.051)
  line L589 (-1.4982, 1.2133) -> (-1.0117, 1.2133)
  line L590 (-1.4982, 1.051) -> (-1.4982, 1.2133)
  line L591 (-1.4982, 1.3765) -> (-1.4982, 1.2133)
  line L592 (-1.4982, 1.2133) -> (-1.6598, 1.2133)
  line L593 (-2.1407, 1.5386) -> (-1.9819, 1.5386)
  line L594 (-2.1407, 1.3759) -> (-2.1407, 1.5386)
  line L595 (-2.3059, 1.3759) -> (-2.1407, 1.3759)
  line L596 (-1.7642, 2.0832) -> (-1.7642, 2.2076)
  line L597 (-1.7642, 2.2076) -> (-2.1735, 2.2076)
  line L598 (-2.1735, 2.0832) -> (-1.7642, 2.0832)
  line L599 (-1.9819, 1.7042) -> (-2.63, 1.7042)
  line L600 (-2.4679, 1.5386) -> (-2.3059, 1.5386)
  line L601 (-2.3059, 1.5386) -> (-2.3059, 1.3759)
  line L602 (-1.9819, 1.5386) -> (-1.9819, 1.7042)
  line L603 (-1.6598, 1.7042) -> (-1.8224, 1.7042)
  line L604 (-1.9819, 1.5386) -> (-1.8224, 1.5386)
  line L605 (-1.8224, 1.7042) -> (-1.8224, 1.5386)
  line L606 (-1.8224, 1.5386) -> (-1.6598, 1.5386)
  line L607 (-2.1735, 2.2076) -> (-2.1735, 2.0832)
  line L608 (-2.1735, 2.2076) -> (-2.1735, 2.3469)
  line L609 (-2.3073, 2.3469) -> (-2.3073, 2.2076)
  line L610 (-2.1735, 2.3469) -> (-2.3073, 2.3469)
  line L611 (-2.4465, 2.2076) -> (-2.5758, 2.2076)
  line L612 (-2.4465, 2.4776) -> (-2.4465, 2.2076)
  line L613 (-2.5758, 2.2076) -> (-2.5758, 2.4776)
  line L614 (-2.3073, 2.2076) -> (-2.1735, 2.2076)
  line L615 (-0.6864, 1.3765) -> (-0.6864, 1.5386)
  line L616 (-0.6864, 1.3765) -> (-0.5216, 1.3765)
  line L617 (-0.5216, 1.7042) -> (-0.5216, 1.5386)
  line L618 (-0.2017, 1.2144) -> (-0.2017, 1.0574)
  line L619 (-0.2017, 1.0574) -> (-0.5216, 1.0574)
  line L620 (-0.3615, 1.2144) -> (-0.2017, 1.2144)
  line L621 (0.1158, 1.2144) -> (-0.0419, 1.2144)
  line L622 (-0.5216, 1.0574) -> (-0.5216, 1.3765)
  line L623 (-0.3615, 1.3765) -> (-0.3615, 1.2144)
  line L624 (-0.0419, 1.2144) -> (-0.0419, 1.3765)
  line L625 (-0.0419, 1.3765) -> (-0.3615, 1.3765)
  line L626 (-0.5216, 1.5386) -> (0.1158, 1.5386)
  line L627 (0.1158, 1.5386) -> (0.1158, 1.2144)
  line L628 (-1.6598, 1.5386) -> (-1.6598, 1.3765)
  line L629 (-1.6598, 1.3765) -> (-1.4982, 1.3765)
  line L630 (-1.6598, 1.5386) -> (-1.6598, 1.7042)
  line L631 (-1.0117, 1.5386) -> (-1.6598, 1.5386)
  line L632 (-1.0117, 1.5386) -> (-1.0117, 1.7042)
  line L633 (-0.6864, 1.5386) -> (-1.0117, 1.5386)
  line L634 (-1.0117, 1.7042) -> (-0.5216, 1.7042)
  line L635 (-1.3285, 2.4798) -> (-1.0789, 2.4798)
  line L636 (-1.3285, 2.2176) -> (-1.3285, 2.0832)
  line L637 (-1.3285, 2.2176) -> (-1.3285, 2.0832)
  line L638 (-1.7642, 2.8765) -> (-1.6349, 2.8765)
  line L639 (-1.7642, 2.6098) -> (-1.7642, 2.8765)
  line L640 (-1.6349, 2.6098) -> (-1.7642, 2.6098)
  line L641 (-1.6349, 2.8765) -> (-1.6349, 2.6098)
  line L642 (-2.1735, 2.8765) -> (-1.7642, 2.8765)
  line L643 (-1.7642, 2.8765) -> (-1.7642, 3.0109)
  line L644 (-1.7642, 3.0109) -> (-2.1735, 3.0109)
  line L645 (-2.3073, 2.7372) -> (-2.1735, 2.7372)
  line L646 (-2.3073, 2.8765) -> (-2.3073, 2.7372)
  line L647 (-2.1735, 2.8765) -> (-2.3073, 2.8765)
  line L648 (-2.1735, 3.0109) -> (-2.1735, 2.8765)
  line L649 (-2.1735, 2.7372) -> (-2.1735, 2.8765)
  line L650 (-1.4684, 2.0832) -> (-1.4684, 3.0109)
  line L651 (-1.3285, 2.8765) -> (-1.3285, 2.0832)
  line L652 (-1.3285, 2.0832) -> (-1.4684, 2.0832)
  line L653 (-1.3285, 3.0109) -> (-1.3285, 2.8765)
  line L654 (-1.4684, 3.0109) -> (-1.3285, 3.0109)
  line L655 (-1.3285, 2.6143) -> (-1.3285, 2.4798)
  line L656 (-1.0789, 2.4798) -> (-1.0789, 2.6143)
  line L657 (-1.0789, 2.6143) -> (-1.3285, 2.6143)
  line L658 (-1.3285, 2.6143) -> (-1.3285, 2.4798)
  line L659 (-1.3285, 2.0832) -> (-0.7944, 2.0832)
  line L660 (-0.7944, 2.0832) -> (-0.7944, 2.2176)
  line L661 (-0.7944, 2.2176) -> (-1.3285, 2.2176)
  line L662 (-1.3285, 3.0109) -> (-1.3285, 2.8765)
  line L663 (-1.3285, 2.8765) -> (-0.7944, 2.8765)
  line L664 (-0.7944, 3.0109) -> (-1.3285, 3.0109)
  line L665 (-0.7944, 2.8765) -> (-0.7944, 3.0109)
  line L666 (-0.4968, 2.0832) -> (0.0373, 2.0832)
  line L667 (0.0373, 2.2176) -> (-0.4968, 2.2176)
  line L668 (0.0373, 2.0832) -> (0.0373, 2.2176)
  line L669 (-0.4968, 2.0832) -> (-0.6366, 2.0832)
  line L670 (-0.4968, 2.2176) -> (-0.4968, 2.0832)
  line L671 (-0.4968, 2.8765) -> (-0.4968, 2.0832)
  line L672 (-0.4968, 3.0109) -> (-0.4968, 2.8765)
  line L673 (-0.6366, 2.0832) -> (-0.6366, 3.0109)
  line L674 (-0.6366, 3.0109) -> (-0.4968, 3.0109)
  line L675 (-0.4968, 2.2176) -> (-0.4968, 2.0832)
  line L676 (0.2054, 2.0832) -> (0.2054, 2.7448)
  line L677 (0.3452, 2.0832) -> (0.2054, 2.0832)
  line L678 (0.3452, 2.3476) -> (0.3452, 2.6104)
  line L679 (0.3452, 2.3476) -> (0.3452, 2.0832)
  line L680 (0.4781, 2.3476) -> (0.3452, 2.3476)
  line L681 (0.4781, 2.3476) -> (0.6129, 2.3476)
  line L682 (0.7416, 2.4768) -> (0.3452, 2.4768)
  line L683 (0.6129, 2.3476) -> (0.7416, 2.3476)
  line L684 (0.7416, 2.078) -> (0.7416, 2.3476)
  line L685 (0.8808, 2.743) -> (0.8808, 2.078)
  line L686 (0.8808, 2.078) -> (0.7416, 2.078)
  line L687 (0.7416, 2.3476) -> (0.7416, 2.6051)
  line L688 (0.7416, 2.743) -> (0.8808, 2.743)
  line L689 (0.7416, 2.6051) -> (0.7416, 2.743)
  line L690 (0.3452, 2.7448) -> (0.2054, 2.7448)
  line L691 (0.3452, 2.6104) -> (0.3452, 2.7448)
  line L692 (0.7416, 2.743) -> (0.61, 2.743)
  line L693 (0.3452, 2.7448) -> (0.4717, 2.7448)
  line L694 (0.7416, 2.743) -> (0.7416, 2.8781)
  line L695 (0.61, 2.8781) -> (0.7416, 2.8781)
  line L696 (0.61, 2.743) -> (0.61, 2.8781)
  line L697 (0.4717, 2.7448) -> (0.4717, 2.8781)
  line L698 (0.4717, 2.8781) -> (0.61, 2.8781)
  line L699 (0.3452, 2.8781) -> (0.4717, 2.8781)
  line L700 (0.3452, 2.7448) -> (0.3452, 2.8781)
  line L701 (0.61, 2.8781) -> (0.61, 3.0174)
  line L702 (0.61, 3.0174) -> (0.4717, 3.0174)
  line L703 (0.4717, 3.0174) -> (0.4717, 2.8781)
  line L704 (-1.7642, 2.4776) -> (-1.8967, 2.4776)
  line L705 (-1.7642, 2.2076) -> (-1.7642, 2.4776)
  line L706 (-1.8967, 2.6104) -> (-1.7642, 2.6104)
  line L707 (-1.8967, 2.6104) -> (-1.8967, 2.4776)
  line L708 (-1.7642, 2.6104) -> (-1.7642, 2.4776)
  line L709 (-1.6349, 2.2076) -> (-1.7642, 2.2076)
  line L710 (-1.6349, 2.4776) -> (-1.6349, 2.2076)
  line L711 (-1.7642, 2.4776) -> (-1.6349, 2.4776)
  point P0 (-2.2326, -0.0258)
  constraints: 1426 end point, 310 perpendicular, 186 point on line, 176 parallel, 110 horizontal, 25 vertical, 2 collinear
extrude "Extrusion29" add sketch "Sketch17" along normal blind 0.001 contours L11 L129 L130 L135 L133 L132 L131 L54 L46 L50 L47 L168 L167 L166 L165 L164 L229 L227 L228 L230 L252 L156 L154 L155 L159 L157 L153 L148 L145 L146 L147 L102 L100 L99 L101 L103 L137 L143 L208 L207 L210 L218 L15 L142 L90 L89 L4 L6 L8 L7 L348 L347 L350 L12 L13 | L529 L524 L522 L134 | L121 L486 L485 L484 | L501 L499 L498 L500 | L632 L634 L617 L626 L627 L621 L624 L625 L623 L620 L618 L619 L622 L616 L615 L633 | L590 L585 L584 L592 | L631 L575 L589 L591 L629 L628 | L605 L603 L630 L606 | L567 L566 L569 L368 L599 L602 L593 L594 L595 L601 L600 L369 L562 L561 L563 L564 | L201 L199 L198 L204 L205 L206 | L224 L226 L225 L223 | L197 L200 L203 L202 | L232 L234 L233 L231 | L254 L258 L257 L256 L255 L253 | L264 L267 L269 L270 L268 L266 | L281 L279 L280 L282 | L415 L426 L384 L392 L383 L382 L419 L430 L431 L424 L416 L414 | L364 L365 L366 L367 | L530 L533 L523 L532 | L478 L526 L528 L527 | L482 L477 L480 L481 | L351 L359 L358 L303 L298 L387 L299 L349 L69 L67 L68 L70 L74 L75 L391 L393 L390 L388 L389 L386 L385 L307 L301 L302 L300 L356 L315 L316 L319 L320 L380 L379 L376 L373 L371 L363 L370 L378 L317 L318 L310 L321 L309 L308 L362 L355 L571 L570 L572 L483 L574 L573 L565 L360 | L353 L361 L354 L352 | L184 L120 L487 L492 L125 L491 L490 L489 L506 L505 L513 L508 L507 L128 L122 L183 L188 L185 | L195 L173 L179 L176 L175 L196 L189 L190 L191 L187 L186 L192 L193 L194 | L136 L139 L141 L140 | L171 L172 L170 L182 L181 L180 L178 L177 L174 L169 | L105 L45 L42 L43 L44 L91 | L510 L512 L511 L509 | L138 L110 L111 L109 L107 L108 L39 L36 L37 L32 L35 L106 | L32 L31 L30 L45 | L488 L494 L495 L493 | L514 L515 L516 L519 L521 L520 | L504 L496 L497 L503 L559 L502 L535 L534 L536 L525 L531 L560 L548 L549 L479 L568 L586 L588 L547 L576 L577 L581 L580 L579 L556 L538 L539 L578 L540 L543 L544 L545 L546 L542 L541 L537 L518 L517 | L33 L34 L29 L41 L30 L31 | L104 L113 L119 L118 L116 L115 | L95 L97 L96 L93 | L102 L98 L149 L150 L148 L153 L157 L158 L151 L152 L94 L114 L96 L97 | L114 L283 L117 L112 | L147 L146 L145 L144 | L94 L152 L151 L162 L163 L263 L272 L265 L271 L259 L277 L276 L275 L273 L274 L278 L294 L293 L288 L286 L285 L284 | L157 L160 L161 L158 | L583 L604 L587 L582 | L16 L63 L64 L61 L60 L59 L66 L57 L55 L56 L65 L62 L38 L22 L21 L17 L19 L20 L27 L28 L26 L18 | L23 L24 L76 L25 | L40 L72 L71 L73 | L58 L417 L418 L381 | L77 L82 L83 L79 | L80 L88 L87 L84 | L219 L222 L221 L220 | L235 L238 L237 L236 | L239 L241 L250 L245 | L242 L244 L249 L247 | L251 L261 L260 L262 | L328 L338 L327 L326 | L332 L330 L337 L336 | L333 L335 L334 L331 | L341 L339 L340 L342 | L345 L344 L343 L346 | L322 L325 L329 L324 | L323 L612 L611 L613 | L409 L401 L403 L399 L412 L411 L410 L413 | L396 L398 L397 L406 | L394 L400 L404 L402 L405 L407 L395 L408 | L420 L421 L422 L423 | L425 L429 L428 L427 | L432 L437 L438 L436 | L441 L442 L443 L435 L434 | L446 L447 L453 L452 L456 L455 L454 L451 L450 L449 L448 L445 | L460 L465 L466 L464 | L476 L472 L470 L471 | L469 L474 L475 L473 | L463 L462 L468 L458 | L457 L461 L459 L467 | L550 L551 L555 L554 | L598 L607 L597 L596 | L614 L609 L610 L608 | L649 L645 L646 L647 | L642 L648 L644 L643 | L639 L638 L641 L640 | L704 L707 L706 L708 | L705 L711 L710 L709 | L651 L657 L656 L635 | L651 L636 L652 L650 L654 L653 | L661 L660 L659 L636 | L653 L664 L665 L663 | L670 L667 L668 L666 | L669 L673 L674 L672 L671 L670 | L676 L690 L691 L678 L679 L677 | L700 L699 L697 L693 | L678 L682 L687 L683 L681 L680 | L703 L702 L701 L698 | L687 L689 L688 L685 L686 L684 | L695 L694 L692 L696
sketch "Sketch22" plane through (0, 0, 0.6) normal (0, 0, 1) x (1, 0, 0)
  line L0 (4.9253, 1.0689) -> (6.6212, 1.0689)
  line L1 (6.6212, 1.0689) -> (6.6212, -2.2077)
  line L2 (6.6212, -2.2077) -> (4.9253, -2.2077)
  line L3 (4.9253, -2.2077) -> (4.9253, 1.0689)
  line L4 (4.8939, 1.1056) -> (6.6526, 1.1056)
  line L5 (6.6526, 1.1056) -> (6.6526, 0.6397)
  line L6 (6.6526, 0.6397) -> (4.8939, 0.6397)
  line L7 (4.8939, 0.6397) -> (4.8939, 1.1056)
  line L8 (4.8939, -1.7733) -> (6.6526, -1.7733)
  line L9 (6.6526, -1.7733) -> (6.6526, -2.2391)
  line L10 (6.6526, -2.2391) -> (4.8939, -2.2391)
  line L11 (4.8939, -2.2391) -> (4.8939, -1.7733)
  point P0 (0, 0)
  constraints: 24 end point, 6 parallel, 3 horizontal, 3 perpendicular